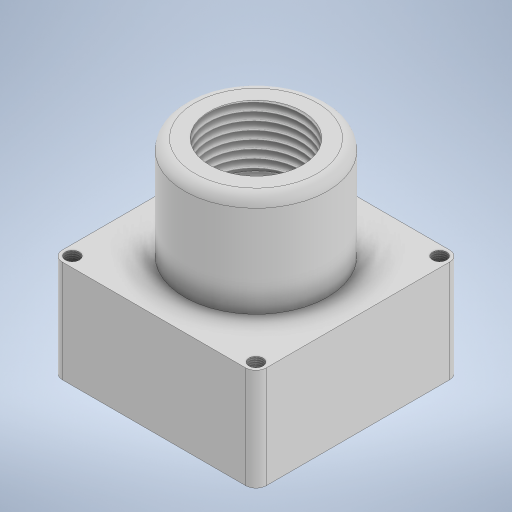
# Autodesk Inventor part: Practica1Inventor
Saved by Autodesk Inventor 2024 (Build 280153000, 153)
## iProperties
Created: 2024-02-18
Part Number: Practica1Inventor
Material: Genérico
Document SubType Name: Modeling
Designer: Gregorio
Density: 1 g/cm^3
Appearance: Valor por defecto
Author: Gregorio
Autodesk Inventor part; units mm, degrees
ref_plane "YZ Plane" through (0, 0, 0) normal (1, 0, 0) x (0, 1, 0)
ref_plane "XZ Plane" through (0, 0, 0) normal (0, 1, 0) x (-1, 0, 0)
ref_plane "XY Plane" through (0, 0, 0) normal (0, 0, 1) x (1, 0, 0)
sketch "Boceto1" plane through (0, 0, 0) normal (0, 1, 0) x (-1, 0, 0)
  line L0 (50, 50) -> (-50, 50)
  line L1 (-50, 50) -> (-50, -50)
  line L2 (-50, -50) -> (50, -50)
  line L3 (50, -50) -> (50, 50)
  line L4 (50, 50) -> (-50, -50) construction
  line L5 (-50, 50) -> (50, -50) construction
  point P0 (0, 0)
  dimension "d0" = 100
  dimension "d1" = 100
  constraints: 12 end point, 2 midpoint, 2 parallel, 1 horizontal, 1 perpendicular
  measures "d0" distance of L2.end L1.end
  measures "d1" distance of L0.end L1.end
sketch "Boceto2" plane through (0, 0, 0) normal (0, 1, 0) x (-1, 0, 0)
  point P0 (0, 0)
extrude "Extrusión1" add sketch "Boceto1" along normal blind 50
sketch "Boceto3" plane through (0, 50, 0) normal (0, 1, 0) x (1, 0, 0)
  line L0 (-50, 50) -> (-50, -50) projected
  line L1 (50, 50) -> (-50, 50) projected
  line L2 (50, -50) -> (50, 50) projected
  line L3 (-50, -50) -> (50, -50) projected
  point P0 (0, 0)
  point P1 (-45, -45)
  point P2 (-45, 45)
  point P3 (45, 45)
  point P4 (45, -45)
  dimension "d11" = 5
  dimension "d12" = 5
  dimension "d13" = 5
  dimension "d14" = 5
  dimension "d15" = 5
  dimension "d16" = 5
  dimension "d17" = 5
  dimension "d18" = 5
  measures "d11" distance from line of L0 point (-45, 45)
  measures "d12" distance from line of L1 point (-45, 45)
  measures "d13" distance from line of L2 point (45, 45)
  measures "d14" distance from line of L1 point (45, 45)
  measures "d15" distance from line of L3 point (-45, -45)
  measures "d16" distance from line of L0 point (-45, -45)
  measures "d17" distance from line of L3 point (45, -45)
  measures "d18" distance from line of L2 point (45, -45)
hole "Agujero1" at (-45, 50, 45) at (-45, 50, -45) at (45, 50, -45) at (45, 50, 45) direction (0, -1, 0) diameter 6.917 end through all counterbore diameter 8 counterbore depth 0 thread size "M8x1" class "6H" standard "ANSI Metric M Profile"
fillet "Empalme1" radius 5 4 edges at (-50, 25, 50) (50, 25, 50) (50, 25, -50) (-50, 25, -50)
sketch "Boceto4" plane through (0, 50, 0) normal (0, 1, 0) x (1, 0, 0)
  point P0 (0, 0)
sketch "Boceto5" plane through (0, 50, 0) normal (0, 1, 0) x (1, 0, 0)
  circle A0 centre (0, 0) radius 35
  dimension "d20" = 70
  constraints: 1 centre point, 1 coincident
  measures "d20" diameter of A0
extrude "Extrusión2" add sketch "Boceto5" along normal blind 50
fillet "Empalme2" radius 5 1 edges at (-35, 100, 0)
sketch "Boceto7" plane through (0, 100, 0) normal (0, 1, 0) x (1, 0, 0)
  point P0 (0, 0)
hole "Agujero3" at (0, 100, 0) direction (0, -1, 0) diameter 45.6699 depth 30 counterbore diameter 50 counterbore depth 0 thread size "M50x4" class "6H" standard "ANSI Metric M Profile"
